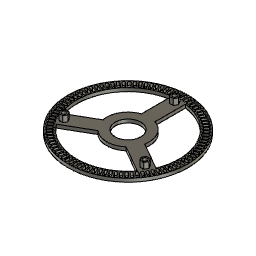
front_speed_sensor_disc (Autodesk Fusion 360 design; units mm, degrees)
Autodesk Fusion 360 part; units mm, degrees
(part 1 of 2)
sketch "Sketch6" plane through (0, 0, 0) normal (0, 0, 1) x (1, 0, 0)
  circle A0 centre (0, 0) radius 60
  circle A1 centre (0, 0) radius 70
  line L0 (0, 0) -> (0, 60)
  circle A2 centre (0, 54.75) radius 2.45
  line L1 (2.2805, 50.8) -> (4.5611, 54.75)
  line L2 (4.5611, 54.75) -> (2.2805, 58.7)
  line L3 (2.2805, 58.7) -> (-2.2805, 58.7)
  line L4 (-2.2805, 58.7) -> (-4.5611, 54.75)
  line L5 (-4.5611, 54.75) -> (-2.2805, 50.8)
  line L6 (-2.2805, 50.8) -> (2.2805, 50.8)
  circle A3 centre (0, 0) radius 9.55 construction
  circle A4 centre (0, 0) radius 7.4 construction
  circle A5 centre (0, 0) radius 15
  line L7 (0, 60) -> (0, 70)
  circle A6 centre (0, 67.5) radius 1.5
  circle A7 centre (0, 62.5) radius 1.5
  line L8 (-1.5, 67.5) -> (-1.5, 62.5)
  line L9 (1.5, 67.5) -> (1.5, 62.5)
  line L10 (0, 67.5) -> (0, 62.5)
  line L11 (-8, 59.4643) -> (-8, 12.6886)
  line L12 (8, 59.4643) -> (8, 12.6886)
  line L13 (-6.2049, 67.2309) -> (-5.8561, 62.2431)
  line L14 (-3.2122, 67.4402) -> (-2.8634, 62.4524)
  line L15 (-4.7086, 67.3356) -> (-4.3598, 62.3478)
  circle A8 centre (-4.3598, 62.3478) radius 1.5
  line L16 (-4.1854, 59.8538) -> (-4.883, 69.8295)
  circle A9 centre (-4.7086, 67.3356) radius 1.5
  line L17 (-10.8796, 66.6343) -> (-10.1837, 61.683)
  line L18 (-7.9088, 67.0519) -> (-7.2129, 62.1005)
  line L19 (-9.3942, 66.8431) -> (-8.6983, 61.8918)
  circle A10 centre (-8.6983, 61.8918) radius 1.5
  line L20 (-8.3504, 59.4161) -> (-9.7421, 69.3188)
  circle A11 centre (-9.3942, 66.8431) radius 1.5
  line L21 (-15.5013, 65.7131) -> (-14.4617, 60.8224)
  line L22 (-12.5668, 66.3368) -> (-11.5273, 61.4461)
  line L23 (-14.034, 66.025) -> (-12.9945, 61.1342)
  circle A12 centre (-12.9945, 61.1342) radius 1.5
  line L24 (-12.4747, 58.6889) -> (-14.5538, 68.4703)
  circle A13 centre (-14.034, 66.025) radius 1.5
  line L25 (-20.0474, 64.4717) -> (-18.6692, 59.6654)
  line L26 (-17.1636, 65.2986) -> (-15.7854, 60.4923)
  line L27 (-18.6055, 64.8852) -> (-17.2273, 60.0789)
  circle A14 centre (-17.2273, 60.0789) radius 1.5
  line L28 (-16.5382, 57.6757) -> (-19.2946, 67.2883)
  circle A15 centre (-18.6055, 64.8852) radius 1.5
  line L29 (-24.4959, 62.9162) -> (-22.7858, 58.2178)
  line L30 (-21.6768, 63.9423) -> (-19.9667, 59.2438)
  line L31 (-23.0864, 63.4293) -> (-21.3763, 58.7308)
  circle A16 centre (-21.3763, 58.7308) radius 1.5
  line L32 (-20.5212, 56.3816) -> (-23.9414, 65.7785)
  circle A17 centre (-23.0864, 63.4293) radius 1.5
  line L33 (-28.825, 61.0542) -> (-26.7914, 56.4865)
  line L34 (-26.0844, 62.2744) -> (-24.0507, 57.7067)
  line L35 (-27.4547, 61.6643) -> (-25.421, 57.0966)
  circle A18 centre (-25.421, 57.0966) radius 1.5
  line L36 (-24.4042, 54.8127) -> (-28.4716, 63.9482)
  circle A19 centre (-27.4547, 61.6643) radius 1.5
  line L37 (-33.0138, 58.8948) -> (-30.6664, 54.48)
  line L38 (-30.3649, 60.3032) -> (-28.0176, 55.8884)
  line L39 (-31.6893, 59.599) -> (-29.342, 55.1842)
  circle A20 centre (-29.342, 55.1842) radius 1.5
  line L40 (-28.1683, 52.9769) -> (-32.863, 61.8063)
  circle A21 centre (-31.6893, 59.599) radius 1.5
  line L41 (-37.0416, 56.4484) -> (-34.392, 52.2081)
  line L42 (-34.4975, 58.0381) -> (-31.8479, 53.7979)
  line L43 (-35.7696, 57.2432) -> (-33.12, 53.003)
  circle A22 centre (-33.12, 53.003) radius 1.5
  line L44 (-31.7952, 50.8829) -> (-37.0943, 59.3634)
  circle A23 centre (-35.7696, 57.2432) radius 1.5
  line L45 (-40.889, 53.727) -> (-37.9501, 49.6819)
  line L46 (-38.462, 55.4903) -> (-35.5231, 51.4452)
  line L47 (-39.6755, 54.6086) -> (-36.7366, 50.5636)
  circle A24 centre (-36.7366, 50.5636) radius 1.5
  line L48 (-35.2671, 48.541) -> (-41.145, 56.6312)
  circle A25 centre (-39.6755, 54.6086) radius 1.5
  line L49 (-44.5372, 50.7438) -> (-41.3233, 46.9136)
  line L50 (-42.2391, 52.6722) -> (-39.0252, 48.842)
  line L51 (-43.3882, 51.708) -> (-40.1742, 47.8778)
  circle A26 centre (-40.1742, 47.8778) radius 1.5
  line L52 (-38.5673, 45.9627) -> (-44.9951, 53.6231)
  circle A27 centre (-43.3882, 51.708) radius 1.5
  line L53 (-47.9684, 47.5134) -> (-44.4952, 43.9167)
  line L54 (-45.8104, 49.5974) -> (-42.3371, 46.0007)
  line L55 (-46.8894, 48.5554) -> (-43.4161, 44.9587)
  circle A28 centre (-43.4161, 44.9587) radius 1.5
  line L56 (-41.6795, 43.1604) -> (-48.6261, 50.3538)
  circle A29 centre (-46.8894, 48.5554) radius 1.5
  line L57 (-51.166, 44.0516) -> (-47.4502, 40.7059)
  line L58 (-49.1586, 46.281) -> (-45.4429, 42.9354)
  line L59 (-50.1623, 45.1663) -> (-46.4466, 41.8207)
  circle A30 centre (-46.4466, 41.8207) radius 1.5
  line L60 (-44.5887, 40.1478) -> (-52.0201, 46.8391)
  circle A31 centre (-50.1623, 45.1663) radius 1.5
  line L61 (-54.1142, 40.3751) -> (-50.1742, 37.2968)
  line L62 (-52.2672, 42.7392) -> (-48.3272, 39.6609)
  line L63 (-53.1907, 41.5571) -> (-49.2507, 38.4788)
  circle A32 centre (-49.2507, 38.4788) radius 1.5
  line L64 (-47.2806, 36.9397) -> (-55.1608, 43.0963)
  circle A33 centre (-53.1907, 41.5571) radius 1.5
  line L65 (-56.7988, 36.502) -> (-52.6536, 33.706)
  line L66 (-55.1212, 38.9891) -> (-50.9761, 36.1931)
  line L67 (-55.96, 37.7455) -> (-51.8148, 34.9496)
  circle A34 centre (-51.8148, 34.9496) radius 1.5
  line L68 (-49.7423, 33.5516) -> (-58.0326, 39.1435)
  circle A35 centre (-55.96, 37.7455) radius 1.5
  line L69 (-59.2067, 32.451) -> (-54.8766, 29.951)
  line L70 (-57.7067, 35.049) -> (-53.3766, 32.549)
  line L71 (-58.4567, 33.75) -> (-54.1266, 31.25)
  circle A36 centre (-54.1266, 31.25) radius 1.5
  line L72 (-51.9615, 30) -> (-60.6218, 35)
  circle A37 centre (-58.4567, 33.75) radius 1.5
  line L73 (-61.3262, 28.2419) -> (-56.8322, 26.05)
  line L74 (-60.011, 30.9382) -> (-55.5171, 28.7464)
  line L75 (-60.6686, 29.5901) -> (-56.1746, 27.3982)
  circle A38 centre (-56.1746, 27.3982) radius 1.5
  line L76 (-53.9276, 26.3023) -> (-62.9156, 30.686)
  circle A39 centre (-60.6686, 29.5901) radius 1.5
  line L77 (-63.1468, 23.8952) -> (-58.5109, 22.0221)
  line L78 (-62.023, 26.6767) -> (-57.3871, 24.8037)
  line L79 (-62.5849, 25.2859) -> (-57.949, 23.4129)
  circle A40 centre (-57.949, 23.4129) radius 1.5
  line L80 (-55.631, 22.4764) -> (-64.9029, 26.2225)
  circle A41 centre (-62.5849, 25.2859) radius 1.5
  line L81 (-64.6598, 19.4321) -> (-59.9046, 17.887)
  line L82 (-63.7328, 22.2852) -> (-58.9775, 20.7401)
  line L83 (-64.1963, 20.8586) -> (-59.441, 19.3136)
  circle A42 centre (-59.441, 19.3136) radius 1.5
  line L84 (-57.0634, 18.541) -> (-66.574, 21.6312)
  circle A43 centre (-64.1963, 20.8586) radius 1.5
  line L85 (-65.8578, 14.8743) -> (-61.0064, 13.6647)
  line L86 (-65.1321, 17.7852) -> (-60.2806, 16.5756)
  line L87 (-65.495, 16.3297) -> (-60.6435, 15.1201)
  circle A44 centre (-60.6435, 15.1201) radius 1.5
  line L88 (-58.2177, 14.5153) -> (-67.9207, 16.9345)
  circle A45 centre (-65.495, 16.3297) radius 1.5
  line L89 (-66.735, 10.244) -> (-61.811, 9.3758)
  line L90 (-66.2141, 13.1985) -> (-61.29, 12.3302)
  line L91 (-66.4745, 11.7213) -> (-61.5505, 10.853)
  circle A46 centre (-61.5505, 10.853) radius 1.5
  line L92 (-59.0885, 10.4189) -> (-68.9365, 12.1554)
  circle A47 centre (-66.4745, 11.7213) radius 1.5
  line L93 (-67.287, 5.5639) -> (-62.3144, 5.0412)
  line L94 (-66.9734, 8.5475) -> (-62.0008, 8.0248)
  line L95 (-67.1302, 7.0557) -> (-62.1576, 6.533)
  circle A48 centre (-62.1576, 6.533) radius 1.5
  line L96 (-59.6713, 6.2717) -> (-69.6165, 7.317)
  circle A49 centre (-67.1302, 7.0557) radius 1.5
  line L97 (-67.5112, 0.8566) -> (-62.5143, 0.6821)
  line L98 (-67.4065, 3.8548) -> (-62.4096, 3.6803)
  line L99 (-67.4589, 2.3557) -> (-62.4619, 2.1812)
  circle A50 centre (-62.4619, 2.1812) radius 1.5
  line L100 (-59.9634, 2.094) -> (-69.9574, 2.443)
  circle A51 centre (-67.4589, 2.3557) radius 1.5
  line L101 (-67.4065, -3.8548) -> (-62.4096, -3.6803)
  line L102 (-67.5112, -0.8566) -> (-62.5143, -0.6821)
  line L103 (-67.4589, -2.3557) -> (-62.4619, -2.1812)
  circle A52 centre (-62.4619, -2.1812) radius 1.5
  line L104 (-59.9634, -2.094) -> (-69.9574, -2.443)
  circle A53 centre (-67.4589, -2.3557) radius 1.5
  line L105 (-66.9734, -8.5475) -> (-62.0008, -8.0248)
  line L106 (-67.287, -5.5639) -> (-62.3144, -5.0412)
  line L107 (-67.1302, -7.0557) -> (-62.1576, -6.533)
  circle A54 centre (-62.1576, -6.533) radius 1.5
  line L108 (-59.6713, -6.2717) -> (-69.6165, -7.317)
  circle A55 centre (-67.1302, -7.0557) radius 1.5
  line L109 (-66.2141, -13.1985) -> (-61.29, -12.3302)
  line L110 (-66.735, -10.244) -> (-61.811, -9.3758)
  line L111 (-66.4745, -11.7213) -> (-61.5505, -10.853)
  circle A56 centre (-61.5505, -10.853) radius 1.5
  line L112 (-59.0885, -10.4189) -> (-68.9365, -12.1554)
  circle A57 centre (-66.4745, -11.7213) radius 1.5
  line L113 (-65.1321, -17.7852) -> (-60.2806, -16.5756)
  line L114 (-65.8578, -14.8743) -> (-61.0064, -13.6647)
  line L115 (-65.495, -16.3297) -> (-60.6435, -15.1201)
  circle A58 centre (-60.6435, -15.1201) radius 1.5
  line L116 (-58.2177, -14.5153) -> (-67.9207, -16.9345)
  circle A59 centre (-65.495, -16.3297) radius 1.5
  line L117 (-63.7328, -22.2852) -> (-58.9775, -20.7401)
  line L118 (-64.6598, -19.4321) -> (-59.9046, -17.887)
  line L119 (-64.1963, -20.8586) -> (-59.441, -19.3136)
  circle A60 centre (-59.441, -19.3136) radius 1.5
  line L120 (-57.0634, -18.541) -> (-66.574, -21.6312)
  circle A61 centre (-64.1963, -20.8586) radius 1.5
  line L121 (-62.023, -26.6767) -> (-57.3871, -24.8037)
  line L122 (-63.1468, -23.8952) -> (-58.5109, -22.0221)
  line L123 (-62.5849, -25.2859) -> (-57.949, -23.4129)
  circle A62 centre (-57.949, -23.4129) radius 1.5
  line L124 (-55.631, -22.4764) -> (-64.9029, -26.2225)
  circle A63 centre (-62.5849, -25.2859) radius 1.5
  line L125 (-60.011, -30.9382) -> (-55.5171, -28.7464)
  line L126 (-61.3262, -28.2419) -> (-56.8322, -26.05)
  line L127 (-60.6686, -29.5901) -> (-56.1746, -27.3982)
  circle A64 centre (-56.1746, -27.3982) radius 1.5
  line L128 (-53.9276, -26.3023) -> (-62.9156, -30.686)
  circle A65 centre (-60.6686, -29.5901) radius 1.5
  line L129 (-57.7067, -35.049) -> (-53.3766, -32.549)
  line L130 (-59.2067, -32.451) -> (-54.8766, -29.951)
  line L131 (-58.4567, -33.75) -> (-54.1266, -31.25)
  circle A66 centre (-54.1266, -31.25) radius 1.5
  line L132 (-51.9615, -30) -> (-60.6218, -35)
  circle A67 centre (-58.4567, -33.75) radius 1.5
  line L133 (-55.1212, -38.9891) -> (-50.9761, -36.1931)
  line L134 (-56.7988, -36.502) -> (-52.6536, -33.706)
  line L135 (-55.96, -37.7455) -> (-51.8148, -34.9496)
  circle A68 centre (-51.8148, -34.9496) radius 1.5
  line L136 (-49.7423, -33.5516) -> (-58.0326, -39.1435)
  circle A69 centre (-55.96, -37.7455) radius 1.5
  line L137 (-52.2672, -42.7392) -> (-48.3272, -39.6609)
  line L138 (-54.1142, -40.3751) -> (-50.1742, -37.2968)
  line L139 (-53.1907, -41.5571) -> (-49.2507, -38.4788)
  circle A70 centre (-49.2507, -38.4788) radius 1.5
  line L140 (-47.2806, -36.9397) -> (-55.1608, -43.0963)
  circle A71 centre (-53.1907, -41.5571) radius 1.5
  line L141 (-49.1586, -46.281) -> (-45.4429, -42.9354)
  line L142 (-51.166, -44.0516) -> (-47.4502, -40.7059)
  line L143 (-50.1623, -45.1663) -> (-46.4466, -41.8207)
  circle A72 centre (-46.4466, -41.8207) radius 1.5
  line L144 (-44.5887, -40.1478) -> (-52.0201, -46.8391)
  circle A73 centre (-50.1623, -45.1663) radius 1.5
  line L145 (-45.8104, -49.5974) -> (-42.3371, -46.0007)
  line L146 (-47.9684, -47.5134) -> (-44.4952, -43.9167)
  line L147 (-46.8894, -48.5554) -> (-43.4161, -44.9587)
  circle A74 centre (-43.4161, -44.9587) radius 1.5
  line L148 (-41.6795, -43.1604) -> (-48.6261, -50.3538)
  circle A75 centre (-46.8894, -48.5554) radius 1.5
  line L149 (-42.2391, -52.6722) -> (-39.0252, -48.842)
  line L150 (-44.5372, -50.7438) -> (-41.3233, -46.9136)
  line L151 (-43.3882, -51.708) -> (-40.1742, -47.8778)
  circle A76 centre (-40.1742, -47.8778) radius 1.5
  line L152 (-38.5673, -45.9627) -> (-44.9951, -53.6231)
  circle A77 centre (-43.3882, -51.708) radius 1.5
  line L153 (-38.462, -55.4903) -> (-35.5231, -51.4452)
  line L154 (-40.889, -53.727) -> (-37.9501, -49.6819)
  line L155 (-39.6755, -54.6086) -> (-36.7366, -50.5636)
  circle A78 centre (-36.7366, -50.5636) radius 1.5
  line L156 (-35.2671, -48.541) -> (-41.145, -56.6312)
  circle A79 centre (-39.6755, -54.6086) radius 1.5
  line L157 (-34.4975, -58.0381) -> (-31.8479, -53.7979)
  line L158 (-37.0416, -56.4484) -> (-34.392, -52.2081)
  line L159 (-35.7696, -57.2432) -> (-33.12, -53.003)
  circle A80 centre (-33.12, -53.003) radius 1.5
  line L160 (-31.7952, -50.8829) -> (-37.0943, -59.3634)
  circle A81 centre (-35.7696, -57.2432) radius 1.5
  line L161 (-30.3649, -60.3032) -> (-28.0176, -55.8884)
  line L162 (-33.0138, -58.8948) -> (-30.6664, -54.48)
  line L163 (-31.6893, -59.599) -> (-29.342, -55.1842)
  circle A82 centre (-29.342, -55.1842) radius 1.5
  line L164 (-28.1683, -52.9769) -> (-32.863, -61.8063)
  circle A83 centre (-31.6893, -59.599) radius 1.5
  line L165 (-26.0844, -62.2744) -> (-24.0507, -57.7067)
  line L166 (-28.825, -61.0542) -> (-26.7914, -56.4865)
  line L167 (-27.4547, -61.6643) -> (-25.421, -57.0966)
  circle A84 centre (-25.421, -57.0966) radius 1.5
  line L168 (-24.4042, -54.8127) -> (-28.4716, -63.9482)
  circle A85 centre (-27.4547, -61.6643) radius 1.5
  line L169 (-21.6768, -63.9423) -> (-19.9667, -59.2438)
  line L170 (-24.4959, -62.9162) -> (-22.7858, -58.2178)
  line L171 (-23.0864, -63.4293) -> (-21.3763, -58.7308)
  circle A86 centre (-21.3763, -58.7308) radius 1.5
  line L172 (-20.5212, -56.3816) -> (-23.9414, -65.7785)
  circle A87 centre (-23.0864, -63.4293) radius 1.5
  line L173 (-17.1636, -65.2986) -> (-15.7854, -60.4923)
  line L174 (-20.0474, -64.4717) -> (-18.6692, -59.6654)
  line L175 (-18.6055, -64.8852) -> (-17.2273, -60.0789)
  circle A88 centre (-17.2273, -60.0789) radius 1.5
  line L176 (-16.5382, -57.6757) -> (-19.2946, -67.2883)
  circle A89 centre (-18.6055, -64.8852) radius 1.5
  line L177 (-12.5668, -66.3368) -> (-11.5273, -61.4461)
  line L178 (-15.5013, -65.7131) -> (-14.4617, -60.8224)
  line L179 (-14.034, -66.025) -> (-12.9945, -61.1342)
  circle A90 centre (-12.9945, -61.1342) radius 1.5
  line L180 (-12.4747, -58.6889) -> (-14.5538, -68.4703)
  circle A91 centre (-14.034, -66.025) radius 1.5
  line L181 (-7.9088, -67.0519) -> (-7.2129, -62.1005)
  line L182 (-10.8796, -66.6343) -> (-10.1837, -61.683)
  line L183 (-9.3942, -66.8431) -> (-8.6983, -61.8918)
  circle A92 centre (-8.6983, -61.8918) radius 1.5
  line L184 (-8.3504, -59.4161) -> (-9.7421, -69.3188)
  circle A93 centre (-9.3942, -66.8431) radius 1.5
  line L185 (-3.2122, -67.4402) -> (-2.8634, -62.4524)
  line L186 (-6.2049, -67.2309) -> (-5.8561, -62.2431)
  line L187 (-4.7086, -67.3356) -> (-4.3598, -62.3478)
  circle A94 centre (-4.3598, -62.3478) radius 1.5
  line L188 (-4.1854, -59.8538) -> (-4.883, -69.8295)
  circle A95 centre (-4.7086, -67.3356) radius 1.5
  line L189 (1.5, -67.5) -> (1.5, -62.5)
  line L190 (-1.5, -67.5) -> (-1.5, -62.5)
  line L191 (0, -67.5) -> (0, -62.5)
  circle A96 centre (0, -62.5) radius 1.5
  line L192 (0, -60) -> (0, -70)
  circle A97 centre (0, -67.5) radius 1.5
  line L193 (6.2049, -67.2309) -> (5.8561, -62.2431)
  line L194 (3.2122, -67.4402) -> (2.8634, -62.4524)
  line L195 (4.7086, -67.3356) -> (4.3598, -62.3478)
  circle A98 centre (4.3598, -62.3478) radius 1.5
  line L196 (4.1854, -59.8538) -> (4.883, -69.8295)
  circle A99 centre (4.7086, -67.3356) radius 1.5
  line L197 (10.8796, -66.6343) -> (10.1837, -61.683)
  line L198 (7.9088, -67.0519) -> (7.2129, -62.1005)
  line L199 (9.3942, -66.8431) -> (8.6983, -61.8918)
  circle A100 centre (8.6983, -61.8918) radius 1.5
  line L200 (8.3504, -59.4161) -> (9.7421, -69.3188)
  circle A101 centre (9.3942, -66.8431) radius 1.5
  line L201 (15.5013, -65.7131) -> (14.4617, -60.8224)
  line L202 (12.5668, -66.3368) -> (11.5273, -61.4461)
  line L203 (14.034, -66.025) -> (12.9945, -61.1342)
  circle A102 centre (12.9945, -61.1342) radius 1.5
  line L204 (12.4747, -58.6889) -> (14.5538, -68.4703)
  circle A103 centre (14.034, -66.025) radius 1.5
  line L205 (20.0474, -64.4717) -> (18.6692, -59.6654)
  line L206 (17.1636, -65.2986) -> (15.7854, -60.4923)
  line L207 (18.6055, -64.8852) -> (17.2273, -60.0789)
  circle A104 centre (17.2273, -60.0789) radius 1.5
  line L208 (16.5382, -57.6757) -> (19.2946, -67.2883)
  circle A105 centre (18.6055, -64.8852) radius 1.5
  line L209 (24.4959, -62.9162) -> (22.7858, -58.2178)
  line L210 (21.6768, -63.9423) -> (19.9667, -59.2438)
  line L211 (23.0864, -63.4293) -> (21.3763, -58.7308)
  circle A106 centre (21.3763, -58.7308) radius 1.5
  line L212 (20.5212, -56.3816) -> (23.9414, -65.7785)
  circle A107 centre (23.0864, -63.4293) radius 1.5
  line L213 (28.825, -61.0542) -> (26.7914, -56.4865)
  line L214 (26.0844, -62.2744) -> (24.0507, -57.7067)
  line L215 (27.4547, -61.6643) -> (25.421, -57.0966)
  circle A108 centre (25.421, -57.0966) radius 1.5
  line L216 (24.4042, -54.8127) -> (28.4716, -63.9482)
  circle A109 centre (27.4547, -61.6643) radius 1.5
  line L217 (33.0138, -58.8948) -> (30.6664, -54.48)
  line L218 (30.3649, -60.3032) -> (28.0176, -55.8884)
  line L219 (31.6893, -59.599) -> (29.342, -55.1842)
  circle A110 centre (29.342, -55.1842) radius 1.5
  line L220 (28.1683, -52.9769) -> (32.863, -61.8063)
  circle A111 centre (31.6893, -59.599) radius 1.5
  line L221 (37.0416, -56.4484) -> (34.392, -52.2081)
  line L222 (34.4975, -58.0381) -> (31.8479, -53.7979)
  line L223 (35.7696, -57.2432) -> (33.12, -53.003)
  circle A112 centre (33.12, -53.003) radius 1.5
  line L224 (31.7952, -50.8829) -> (37.0943, -59.3634)
  circle A113 centre (35.7696, -57.2432) radius 1.5
  line L225 (40.889, -53.727) -> (37.9501, -49.6819)
  line L226 (38.462, -55.4903) -> (35.5231, -51.4452)
  line L227 (39.6755, -54.6086) -> (36.7366, -50.5636)
  circle A114 centre (36.7366, -50.5636) radius 1.5
  line L228 (35.2671, -48.541) -> (41.145, -56.6312)
  circle A115 centre (39.6755, -54.6086) radius 1.5
  line L229 (44.5372, -50.7438) -> (41.3233, -46.9136)
  line L230 (42.2391, -52.6722) -> (39.0252, -48.842)
  line L231 (43.3882, -51.708) -> (40.1742, -47.8778)
  circle A116 centre (40.1742, -47.8778) radius 1.5
  line L232 (38.5673, -45.9627) -> (44.9951, -53.6231)
  circle A117 centre (43.3882, -51.708) radius 1.5
  line L233 (47.9684, -47.5134) -> (44.4952, -43.9167)
  line L234 (45.8104, -49.5974) -> (42.3371, -46.0007)
  line L235 (46.8894, -48.5554) -> (43.4161, -44.9587)
  circle A118 centre (43.4161, -44.9587) radius 1.5
  line L236 (41.6795, -43.1604) -> (48.6261, -50.3538)
  circle A119 centre (46.8894, -48.5554) radius 1.5
  line L237 (51.166, -44.0516) -> (47.4502, -40.7059)
  line L238 (49.1586, -46.281) -> (45.4429, -42.9354)
  line L239 (50.1623, -45.1663) -> (46.4466, -41.8207)
  circle A120 centre (46.4466, -41.8207) radius 1.5
  line L240 (44.5887, -40.1478) -> (52.0201, -46.8391)
  circle A121 centre (50.1623, -45.1663) radius 1.5
  line L241 (54.1142, -40.3751) -> (50.1742, -37.2968)
  line L242 (52.2672, -42.7392) -> (48.3272, -39.6609)
  line L243 (53.1907, -41.5571) -> (49.2507, -38.4788)
  circle A122 centre (49.2507, -38.4788) radius 1.5
  line L244 (47.2806, -36.9397) -> (55.1608, -43.0963)
  circle A123 centre (53.1907, -41.5571) radius 1.5
  line L245 (56.7988, -36.502) -> (52.6536, -33.706)
  line L246 (55.1212, -38.9891) -> (50.9761, -36.1931)
  line L247 (55.96, -37.7455) -> (51.8148, -34.9496)
  circle A124 centre (51.8148, -34.9496) radius 1.5
  line L248 (49.7423, -33.5516) -> (58.0326, -39.1435)
  circle A125 centre (55.96, -37.7455) radius 1.5
  line L249 (59.2067, -32.451) -> (54.8766, -29.951)
  line L250 (57.7067, -35.049) -> (53.3766, -32.549)
  line L251 (58.4567, -33.75) -> (54.1266, -31.25)
  circle A126 centre (54.1266, -31.25) radius 1.5
  line L252 (51.9615, -30) -> (60.6218, -35)
  circle A127 centre (58.4567, -33.75) radius 1.5
  line L253 (61.3262, -28.2419) -> (56.8322, -26.05)
  line L254 (60.011, -30.9382) -> (55.5171, -28.7464)
  line L255 (60.6686, -29.5901) -> (56.1746, -27.3982)
  circle A128 centre (56.1746, -27.3982) radius 1.5
  line L256 (53.9276, -26.3023) -> (62.9156, -30.686)
  circle A129 centre (60.6686, -29.5901) radius 1.5
  line L257 (63.1468, -23.8952) -> (58.5109, -22.0221)
  line L258 (62.023, -26.6767) -> (57.3871, -24.8037)
  line L259 (62.5849, -25.2859) -> (57.949, -23.4129)
  circle A130 centre (57.949, -23.4129) radius 1.5
  line L260 (55.631, -22.4764) -> (64.9029, -26.2225)
  circle A131 centre (62.5849, -25.2859) radius 1.5
  line L261 (64.6598, -19.4321) -> (59.9046, -17.887)
  line L262 (63.7328, -22.2852) -> (58.9775, -20.7401)
  line L263 (64.1963, -20.8586) -> (59.441, -19.3136)
  circle A132 centre (59.441, -19.3136) radius 1.5
  line L264 (57.0634, -18.541) -> (66.574, -21.6312)
  circle A133 centre (64.1963, -20.8586) radius 1.5
  line L265 (65.8578, -14.8743) -> (61.0064, -13.6647)
  line L266 (65.1321, -17.7852) -> (60.2806, -16.5756)
  line L267 (65.495, -16.3297) -> (60.6435, -15.1201)
  circle A134 centre (60.6435, -15.1201) radius 1.5
  line L268 (58.2177, -14.5153) -> (67.9207, -16.9345)
  circle A135 centre (65.495, -16.3297) radius 1.5
  line L269 (66.735, -10.244) -> (61.811, -9.3758)
  line L270 (66.2141, -13.1985) -> (61.29, -12.3302)
  line L271 (66.4745, -11.7213) -> (61.5505, -10.853)
  circle A136 centre (61.5505, -10.853) radius 1.5
  line L272 (59.0885, -10.4189) -> (68.9365, -12.1554)
  circle A137 centre (66.4745, -11.7213) radius 1.5
  line L273 (67.287, -5.5639) -> (62.3144, -5.0412)
  line L274 (66.9734, -8.5475) -> (62.0008, -8.0248)
  line L275 (67.1302, -7.0557) -> (62.1576, -6.533)
  circle A138 centre (62.1576, -6.533) radius 1.5
  line L276 (59.6713, -6.2717) -> (69.6165, -7.317)
  circle A139 centre (67.1302, -7.0557) radius 1.5
  line L277 (67.5112, -0.8566) -> (62.5143, -0.6821)
  line L278 (67.4065, -3.8548) -> (62.4096, -3.6803)
  line L279 (67.4589, -2.3557) -> (62.4619, -2.1812)
  circle A140 centre (62.4619, -2.1812) radius 1.5
  line L280 (59.9634, -2.094) -> (69.9574, -2.443)
  circle A141 centre (67.4589, -2.3557) radius 1.5
  line L281 (67.4065, 3.8548) -> (62.4096, 3.6803)
  line L282 (67.5112, 0.8566) -> (62.5143, 0.6821)
  line L283 (67.4589, 2.3557) -> (62.4619, 2.1812)
  circle A142 centre (62.4619, 2.1812) radius 1.5
  line L284 (59.9634, 2.094) -> (69.9574, 2.443)
  circle A143 centre (67.4589, 2.3557) radius 1.5
  line L285 (66.9734, 8.5475) -> (62.0008, 8.0248)
  line L286 (67.287, 5.5639) -> (62.3144, 5.0412)
  line L287 (67.1302, 7.0557) -> (62.1576, 6.533)
  circle A144 centre (62.1576, 6.533) radius 1.5
  line L288 (59.6713, 6.2717) -> (69.6165, 7.317)
  circle A145 centre (67.1302, 7.0557) radius 1.5
  line L289 (66.2141, 13.1985) -> (61.29, 12.3302)
  line L290 (66.735, 10.244) -> (61.811, 9.3758)
  line L291 (66.4745, 11.7213) -> (61.5505, 10.853)
  circle A146 centre (61.5505, 10.853) radius 1.5
  line L292 (59.0885, 10.4189) -> (68.9365, 12.1554)
  circle A147 centre (66.4745, 11.7213) radius 1.5
  line L293 (65.1321, 17.7852) -> (60.2806, 16.5756)
  line L294 (65.8578, 14.8743) -> (61.0064, 13.6647)
  line L295 (65.495, 16.3297) -> (60.6435, 15.1201)
  circle A148 centre (60.6435, 15.1201) radius 1.5
  line L296 (58.2177, 14.5153) -> (67.9207, 16.9345)
  circle A149 centre (65.495, 16.3297) radius 1.5
  line L297 (63.7328, 22.2852) -> (58.9775, 20.7401)
  line L298 (64.6598, 19.4321) -> (59.9046, 17.887)
  line L299 (64.1963, 20.8586) -> (59.441, 19.3136)
  circle A150 centre (59.441, 19.3136) radius 1.5
  line L300 (57.0634, 18.541) -> (66.574, 21.6312)
  circle A151 centre (64.1963, 20.8586) radius 1.5
  line L301 (62.023, 26.6767) -> (57.3871, 24.8037)
  line L302 (63.1468, 23.8952) -> (58.5109, 22.0221)
  line L303 (62.5849, 25.2859) -> (57.949, 23.4129)
  circle A152 centre (57.949, 23.4129) radius 1.5
  line L304 (55.631, 22.4764) -> (64.9029, 26.2225)
  circle A153 centre (62.5849, 25.2859) radius 1.5
  line L305 (60.011, 30.9382) -> (55.5171, 28.7464)
  line L306 (61.3262, 28.2419) -> (56.8322, 26.05)
  line L307 (60.6686, 29.5901) -> (56.1746, 27.3982)
  circle A154 centre (56.1746, 27.3982) radius 1.5
  line L308 (53.9276, 26.3023) -> (62.9156, 30.686)
  circle A155 centre (60.6686, 29.5901) radius 1.5
  line L309 (57.7067, 35.049) -> (53.3766, 32.549)
  line L310 (59.2067, 32.451) -> (54.8766, 29.951)
  line L311 (58.4567, 33.75) -> (54.1266, 31.25)
  circle A156 centre (54.1266, 31.25) radius 1.5
  line L312 (51.9615, 30) -> (60.6218, 35)
  circle A157 centre (58.4567, 33.75) radius 1.5
  line L313 (55.1212, 38.9891) -> (50.9761, 36.1931)
  line L314 (56.7988, 36.502) -> (52.6536, 33.706)
  line L315 (55.96, 37.7455) -> (51.8148, 34.9496)
  circle A158 centre (51.8148, 34.9496) radius 1.5
  line L316 (49.7423, 33.5516) -> (58.0326, 39.1435)
  circle A159 centre (55.96, 37.7455) radius 1.5
  line L317 (52.2672, 42.7392) -> (48.3272, 39.6609)
  line L318 (54.1142, 40.3751) -> (50.1742, 37.2968)
  line L319 (53.1907, 41.5571) -> (49.2507, 38.4788)
  circle A160 centre (49.2507, 38.4788) radius 1.5
  line L320 (47.2806, 36.9397) -> (55.1608, 43.0963)
  circle A161 centre (53.1907, 41.5571) radius 1.5
  line L321 (49.1586, 46.281) -> (45.4429, 42.9354)
  line L322 (51.166, 44.0516) -> (47.4502, 40.7059)
  line L323 (50.1623, 45.1663) -> (46.4466, 41.8207)
  circle A162 centre (46.4466, 41.8207) radius 1.5
  line L324 (44.5887, 40.1478) -> (52.0201, 46.8391)
  circle A163 centre (50.1623, 45.1663) radius 1.5
  line L325 (45.8104, 49.5974) -> (42.3371, 46.0007)
  line L326 (47.9684, 47.5134) -> (44.4952, 43.9167)
  line L327 (46.8894, 48.5554) -> (43.4161, 44.9587)
  circle A164 centre (43.4161, 44.9587) radius 1.5
  line L328 (41.6795, 43.1604) -> (48.6261, 50.3538)
  circle A165 centre (46.8894, 48.5554) radius 1.5
  line L329 (42.2391, 52.6722) -> (39.0252, 48.842)
  line L330 (44.5372, 50.7438) -> (41.3233, 46.9136)
  line L331 (43.3882, 51.708) -> (40.1742, 47.8778)
  circle A166 centre (40.1742, 47.8778) radius 1.5
  line L332 (38.5673, 45.9627) -> (44.9951, 53.6231)
  circle A167 centre (43.3882, 51.708) radius 1.5
  line L333 (38.462, 55.4903) -> (35.5231, 51.4452)
  line L334 (40.889, 53.727) -> (37.9501, 49.6819)
  line L335 (39.6755, 54.6086) -> (36.7366, 50.5636)
  circle A168 centre (36.7366, 50.5636) radius 1.5
  line L336 (35.2671, 48.541) -> (41.145, 56.6312)
  circle A169 centre (39.6755, 54.6086) radius 1.5
  line L337 (34.4975, 58.0381) -> (31.8479, 53.7979)
  line L338 (37.0416, 56.4484) -> (34.392, 52.2081)
  line L339 (35.7696, 57.2432) -> (33.12, 53.003)
  circle A170 centre (33.12, 53.003) radius 1.5
  line L340 (31.7952, 50.8829) -> (37.0943, 59.3634)
  circle A171 centre (35.7696, 57.2432) radius 1.5
  line L341 (30.3649, 60.3032) -> (28.0176, 55.8884)
  line L342 (33.0138, 58.8948) -> (30.6664, 54.48)
  line L343 (31.6893, 59.599) -> (29.342, 55.1842)
  circle A172 centre (29.342, 55.1842) radius 1.5
  line L344 (28.1683, 52.9769) -> (32.863, 61.8063)
  circle A173 centre (31.6893, 59.599) radius 1.5
  line L345 (26.0844, 62.2744) -> (24.0507, 57.7067)
  line L346 (28.825, 61.0542) -> (26.7914, 56.4865)
  line L347 (27.4547, 61.6643) -> (25.421, 57.0966)
  circle A174 centre (25.421, 57.0966) radius 1.5
  line L348 (24.4042, 54.8127) -> (28.4716, 63.9482)
  circle A175 centre (27.4547, 61.6643) radius 1.5
  line L349 (21.6768, 63.9423) -> (19.9667, 59.2438)
  line L350 (24.4959, 62.9162) -> (22.7858, 58.2178)
  line L351 (23.0864, 63.4293) -> (21.3763, 58.7308)
  circle A176 centre (21.3763, 58.7308) radius 1.5
  line L352 (20.5212, 56.3816) -> (23.9414, 65.7785)
  circle A177 centre (23.0864, 63.4293) radius 1.5
  line L353 (17.1636, 65.2986) -> (15.7854, 60.4923)
  line L354 (20.0474, 64.4717) -> (18.6692, 59.6654)
  line L355 (18.6055, 64.8852) -> (17.2273, 60.0789)
  circle A178 centre (17.2273, 60.0789) radius 1.5
  line L356 (16.5382, 57.6757) -> (19.2946, 67.2883)
  circle A179 centre (18.6055, 64.8852) radius 1.5
  line L357 (12.5668, 66.3368) -> (11.5273, 61.4461)
  line L358 (15.5013, 65.7131) -> (14.4617, 60.8224)
  line L359 (14.034, 66.025) -> (12.9945, 61.1342)
  circle A180 centre (12.9945, 61.1342) radius 1.5
  line L360 (12.4747, 58.6889) -> (14.5538, 68.4703)
  circle A181 centre (14.034, 66.025) radius 1.5
  line L361 (7.9088, 67.0519) -> (7.2129, 62.1005)
  line L362 (10.8796, 66.6343) -> (10.1837, 61.683)
  line L363 (9.3942, 66.8431) -> (8.6983, 61.8918)
  circle A182 centre (8.6983, 61.8918) radius 1.5
  line L364 (8.3504, 59.4161) -> (9.7421, 69.3188)
  circle A183 centre (9.3942, 66.8431) radius 1.5
  line L365 (3.2122, 67.4402) -> (2.8634, 62.4524)
  line L366 (6.2049, 67.2309) -> (5.8561, 62.2431)
  line L367 (4.7086, 67.3356) -> (4.3598, 62.3478)
  circle A184 centre (4.3598, 62.3478) radius 1.5
  line L368 (4.1854, 59.8538) -> (4.883, 69.8295)
  circle A185 centre (4.7086, 67.3356) radius 1.5
  line L369 (-47.4976, -36.6603) -> (-6.9886, -13.2725)
  line L370 (-55.4976, -22.8039) -> (-14.9886, 0.5839)
  line L371 (0, 0) -> (-51.9615, -30)
  line L372 (-49.6954, -23.425) -> (-51.976, -27.375)
  line L373 (-42.8538, -27.375) -> (-45.1344, -23.425)
  line L374 (-45.1344, -23.425) -> (-49.6954, -23.425)
  line L375 (-51.976, -27.375) -> (-49.6954, -31.325)
  circle A186 centre (-47.4149, -27.375) radius 2.45
  line L376 (-45.1344, -31.325) -> (-42.8538, -27.375)
  line L377 (-49.6954, -31.325) -> (-45.1344, -31.325)
  line L378 (55.4976, -22.8039) -> (14.9886, 0.5839)
  line L379 (47.4976, -36.6603) -> (6.9886, -13.2725)
  line L380 (0, 0) -> (51.9615, -30)
  line L381 (45.1344, -31.325) -> (49.6954, -31.325)
  line L382 (45.1344, -23.425) -> (42.8538, -27.375)
  line L383 (42.8538, -27.375) -> (45.1344, -31.325)
  line L384 (49.6954, -31.325) -> (51.976, -27.375)
  circle A187 centre (47.4149, -27.375) radius 2.45
  line L385 (49.6954, -23.425) -> (45.1344, -23.425)
  line L386 (51.976, -27.375) -> (49.6954, -23.425)
  circle A188 centre (0, 0) radius 25
  point P0 (0, 54.75)
  point P1 (0, 65)
  point P2 (-4.5342, 64.8417)
  point P3 (-9.0463, 64.3674)
  point P4 (-13.5143, 63.5796)
  point P5 (-17.9164, 62.482)
  point P6 (-22.2313, 61.08)
  point P7 (-26.4379, 59.3805)
  point P8 (-30.5157, 57.3916)
  point P9 (-34.4448, 55.1231)
  point P10 (-38.206, 52.5861)
  point P11 (-41.7812, 49.7929)
  point P12 (-45.1528, 46.7571)
  point P13 (-48.3044, 43.4935)
  point P14 (-51.2207, 40.018)
  point P15 (-53.8874, 36.3475)
  point P16 (-56.2917, 32.5)
  point P17 (-58.4216, 28.4941)
  point P18 (-60.267, 24.3494)
  point P19 (-61.8187, 20.0861)
  point P20 (-63.0692, 15.7249)
  point P21 (-64.0125, 11.2871)
  point P22 (-64.6439, 6.7944)
  point P23 (-64.9604, 2.2685)
  point P24 (-64.9604, -2.2685)
  point P25 (-64.6439, -6.7944)
  point P26 (-64.0125, -11.2871)
  point P27 (-63.0692, -15.7249)
  point P28 (-61.8187, -20.0861)
  point P29 (-60.267, -24.3494)
  point P30 (-58.4216, -28.4941)
  point P31 (-56.2917, -32.5)
  point P32 (-53.8874, -36.3475)
  point P33 (-51.2207, -40.018)
  point P34 (-48.3044, -43.4935)
  point P35 (-45.1528, -46.7571)
  point P36 (-41.7812, -49.7929)
  point P37 (-38.206, -52.5861)
  point P38 (-34.4448, -55.1231)
  point P39 (-30.5157, -57.3916)
  point P40 (-26.4379, -59.3805)
  point P41 (-22.2313, -61.08)
  point P42 (-17.9164, -62.482)
  point P43 (-13.5143, -63.5796)
  point P44 (-9.0463, -64.3674)
  point P45 (-4.5342, -64.8417)
  point P46 (0, -65)
  point P47 (4.5342, -64.8417)
  point P48 (9.0463, -64.3674)
  point P49 (13.5143, -63.5796)
  point P50 (17.9164, -62.482)
  point P51 (22.2313, -61.08)
  point P52 (26.4379, -59.3805)
  point P53 (30.5157, -57.3916)
  point P54 (34.4448, -55.1231)
  point P55 (38.206, -52.5861)
  point P56 (41.7812, -49.7929)
  point P57 (45.1528, -46.7571)
  point P58 (48.3044, -43.4935)
  point P59 (51.2207, -40.018)
  point P60 (53.8874, -36.3475)
  point P61 (56.2917, -32.5)
  point P62 (58.4216, -28.4941)
  point P63 (60.267, -24.3494)
  point P64 (61.8187, -20.0861)
  point P65 (63.0692, -15.7249)
  point P66 (64.0125, -11.2871)
  point P67 (64.6439, -6.7944)
  point P68 (64.9604, -2.2685)
  point P69 (64.9604, 2.2685)
  point P70 (64.6439, 6.7944)
  point P71 (64.0125, 11.2871)
  point P72 (63.0692, 15.7249)
  point P73 (61.8187, 20.0861)
  point P74 (60.267, 24.3494)
  point P75 (58.4216, 28.4941)
  point P76 (56.2917, 32.5)
  point P77 (53.8874, 36.3475)
  point P78 (51.2207, 40.018)
  point P79 (48.3044, 43.4935)
  point P80 (45.1528, 46.7571)
  point P81 (41.7812, 49.7929)
  point P82 (38.206, 52.5861)
  point P83 (34.4448, 55.1231)
  point P84 (30.5157, 57.3916)
  point P85 (26.4379, 59.3805)
  point P86 (22.2313, 61.08)
  point P87 (17.9164, 62.482)
  point P88 (13.5143, 63.5796)
  point P89 (9.0463, 64.3674)
  point P90 (4.5342, 64.8417)
  point P91 (-47.4149, -27.375)
  point P92 (47.4149, -27.375)
  dimension "d27" = 7.9
  dimension "d28" = 4.9
  dimension "d29" = 19.1
  dimension "d30" = 14.8
  dimension "d31" = 50.8
  dimension "d32" = 30
  dimension "d33" = 120
  dimension "d34" = 140
  dimension "d36" = 3
  dimension "d37" = 5
  dimension "d38" = 3
  dimension "d39" = 16
  dimension "d40" = 16
  dimension "d42" = 360
  dimension "d44" = 360
  dimension "d45" = 50
  constraint coincident A0.centre A1.centre
  constraint coincident A0 L0.end
  constraint vertical L0
  constraint coincident L0 P0
  constraint coincident P0 A2.centre
  constraint concentric A1 A3
  constraint concentric A3 A4
  constraint horizontal L6
  constraint concentric A1 A5
  constraint coincident A1 L7.end
  constraint parallel L0 L7
  constraint coincident L7 A6.centre
  constraint coincident L7 A7.centre
  constraint coincident A6 L8.start
  constraint coincident A7 L8.end
  constraint tangent A7 L8
  constraint coincident A6 L9.start
  constraint coincident A7 L9.end
  constraint tangent A7 L9
  constraint tangent A6 L9
  constraint tangent A6 L8
  constraint coincident A6.centre L10.start
  constraint coincident A7.centre L10.end
  constraint midpoint L10 P1
  constraint midpoint L7 P1
  constraint coincident A0 L11.start
  constraint coincident A5 L11.end
  constraint vertical L11
  constraint coincident A5 L12.end
  constraint parallel L0 L12
  constraint coincident A0 L12.start
  constraint concentric A4 A188
  measures "d27" distance of L3 L6
  measures "d28" diameter of A2
  measures "d29" diameter of A3
  measures "d30" diameter of A4
  measures "d31" distance of L6 A0.centre
  measures "d32" diameter of A5
  measures "d33" diameter of A0
  measures "d34" diameter of A1
  measures "d36" diameter of A6
  measures "d37" distance of A6.centre A7.centre
  measures "d38" diameter of A7
  measures "d45" diameter of A188
extrude "Extrude5" add sketch "Sketch6" along normal blind 4 contours A0 A1 L277 A140 L280 A141 L282 A142 L284 A143 | A0 A1 L281 A142 L284 A143 L286 A144 L288 A145 | A0 A1 L273 A138 L276 A139 L278 A140 L280 A141 | A0 A1 L285 A144 L288 A145 L290 A146 L292 A147 | A0 A1 L269 A136 L272 A137 L274 A138 L276 A139 | A0 A1 L289 A146 L292 A147 L294 A148 L296 A149 | A0 A1 L265 A134 L268 A135 L270 A136 L272 A137 | A0 A1 L293 A148 L296 A149 L298 A150 L300 A151 | A0 A1 L261 A132 L264 A133 L266 A134 L268 A135 | A0 A1 L297 A150 L300 A151 L302 A152 L304 A153 | A0 A1 L257 A130 L260 A131 L262 A132 L264 A133 | A0 A1 L301 A152 L304 A153 L306 A154 L308 A155 | A0 A1 L253 A128 L256 A129 L258 A130 L260 A131 | A0 A1 L305 A154 L308 A155 L310 A156 L312 A157 | A0 L378 L380 L382 L384 L385 L386 A188 | A0 A1 L309 A156 L312 A157 L314 A158 L316 A159 | A0 A1 L249 A126 L252 A127 L254 A128 L256 A129 | A5 L378 L380 A188 | A5 L12 L378 A188 | A0 A1 L313 A158 L316 A159 L318 A160 L320 A161 | A0 A1 L245 A124 L248 A125 L250 A126 L252 A127 | A0 L379 L380 L381 L382 L383 L384 A188 | A5 L379 L380 A188 | A0 A1 L317 A160 L320 A161 L322 A162 L324 A163 | A0 A1 L241 A122 L244 A123 L246 A124 L248 A125 | L380 L381 L382 L383 L384 A187 | L380 L382 L384 A187 L385 L386 | L0 A5 L12 A188 | A5 L369 L379 A188 | A0 L0 L1 L2 L3 L6 L12 A188 | A0 A1 L321 A162 L324 A163 L326 A164 L328 A165 | L0 A5 L11 A188 | A5 L369 L371 A188 | A0 L369 L371 L373 L375 L376 L377 A188 | A0 A1 L361 A182 L364 A183 L366 A184 L368 A185 | A0 L0 L3 L4 L5 L6 L11 A188 | A0 A1 L325 A164 L328 A165 L330 A166 L332 A167 | A0 A1 L237 A120 L240 A121 L242 A122 L244 A123 | A5 L11 L370 A188 | A5 L370 L371 A188 | A0 A1 L133 A68 L136 A69 L138 A70 L140 A71 | A0 L370 L371 L372 L373 L374 L375 A188 | A0 A1 L357 A180 L360 A181 L362 A182 L364 A183 | A0 A1 L7 A6 A7 L9 L365 A184 L368 A185 | L0 A2 L3 L4 L5 L6 | L0 A2 L1 L2 L3 L6 | A0 A1 L329 A166 L332 A167 L334 A168 L336 A169 | A0 A1 L233 A118 L236 A119 L238 A120 L240 A121 | A0 A1 L129 A66 L132 A67 L134 A68 L136 A69 | A0 A1 L137 A70 L140 A71 L142 A72 L144 A73 | L371 L373 L375 A186 L376 L377 | L371 L372 L373 L374 L375 A186 | A0 A1 L353 A178 L356 A179 L358 A180 L360 A181 | A0 A1 L7 A6 A7 L8 L14 A8 L16 A9 | A0 A1 L13 A8 L16 A9 L18 A10 L20 A11 | A0 A1 L333 A168 L336 A169 L338 A170 L340 A171 | A0 A1 L229 A116 L232 A117 L234 A118 L236 A119 | A0 A1 L125 A64 L128 A65 L130 A66 L132 A67 | A0 A1 L141 A72 L144 A73 L146 A74 L148 A75 | A0 A1 L121 A62 L124 A63 L126 A64 L128 A65 | A0 A1 L349 A176 L352 A177 L354 A178 L356 A179 | A0 A1 L17 A10 L20 A11 L22 A12 L24 A13 | A0 A1 L337 A170 L340 A171 L342 A172 L344 A173 | A0 A1 L225 A114 L228 A115 L230 A116 L232 A117 | A0 A1 L145 A74 L148 A75 L150 A76 L152 A77 | A0 A1 L117 A60 L120 A61 L122 A62 L124 A63 | A0 A1 L345 A174 L348 A175 L350 A176 L352 A177 | A0 A1 L21 A12 L24 A13 L26 A14 L28 A15 | A0 A1 L341 A172 L344 A173 L346 A174 L348 A175 | A0 A1 L221 A112 L224 A113 L226 A114 L228 A115 | A0 A1 L149 A76 L152 A77 L154 A78 L156 A79 | A0 A1 L113 A58 L116 A59 L118 A60 L120 A61 | A0 A1 L25 A14 L28 A15 L30 A16 L32 A17 | A0 A1 L217 A110 L220 A111 L222 A112 L224 A113 | A0 A1 L153 A78 L156 A79 L158 A80 L160 A81 | A0 A1 L109 A56 L112 A57 L114 A58 L116 A59 | A0 A1 L29 A16 L32 A17 L34 A18 L36 A19 | A0 A1 L213 A108 L216 A109 L218 A110 L220 A111 | A0 A1 L157 A80 L160 A81 L162 A82 L164 A83 | A0 A1 L105 A54 L108 A55 L110 A56 L112 A57 | A0 A1 L33 A18 L36 A19 L38 A20 L40 A21 | A0 A1 L209 A106 L212 A107 L214 A108 L216 A109 | A0 A1 L161 A82 L164 A83 L166 A84 L168 A85 | A0 A1 L101 A52 L104 A53 L106 A54 L108 A55 | A0 A1 L37 A20 L40 A21 L42 A22 L44 A23 | A0 A1 L205 A104 L208 A105 L210 A106 L212 A107 | A0 A1 L165 A84 L168 A85 L170 A86 L172 A87 | A0 A1 L97 A50 L100 A51 L102 A52 L104 A53 | A0 A1 L41 A22 L44 A23 L46 A24 L48 A25 | A0 A1 L201 A102 L204 A103 L206 A104 L208 A105 | A0 A1 L169 A86 L172 A87 L174 A88 L176 A89 | A0 A1 L93 A48 L96 A49 L98 A50 L100 A51 | A0 A1 L45 A24 L48 A25 L50 A26 L52 A27 | A0 A1 L197 A100 L200 A101 L202 A102 L204 A103 | A0 A1 L173 A88 L176 A89 L178 A90 L180 A91 | A0 A1 L89 A46 L92 A47 L94 A48 L96 A49 | A0 A1 L49 A26 L52 A27 L54 A28 L56 A29 | A0 A1 L193 A98 L196 A99 L198 A100 L200 A101 | A0 A1 L177 A90 L180 A91 L182 A92 L184 A93 | A0 A1 L85 A44 L88 A45 L90 A46 L92 A47 | A0 A1 L53 A28 L56 A29 L58 A30 L60 A31 | A0 A1 L189 A96 L192 A97 L194 A98 L196 A99 | A0 A1 L181 A92 L184 A93 L186 A94 L188 A95 | A0 A1 L81 A42 L84 A43 L86 A44 L88 A45 | A0 A1 L57 A30 L60 A31 L62 A32 L64 A33 | A0 A1 L185 A94 L188 A95 L190 A96 L192 A97 | A0 A1 L77 A40 L80 A41 L82 A42 L84 A43 | A0 A1 L61 A32 L64 A33 L66 A34 L68 A35 | A0 A1 L73 A38 L76 A39 L78 A40 L80 A41 | A0 A1 L65 A34 L68 A35 L70 A36 L72 A37 | A0 A1 L69 A36 L72 A37 L74 A38 L76 A39